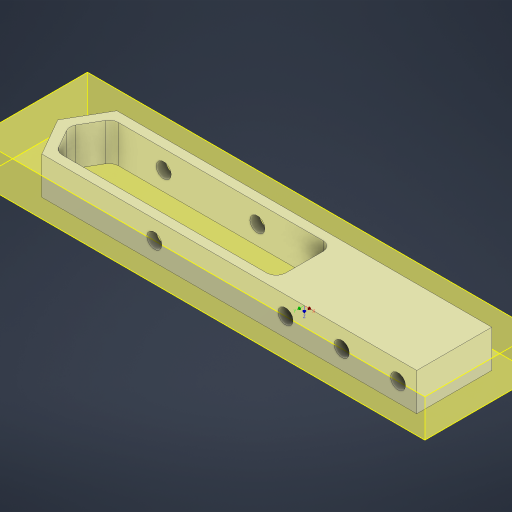
# Autodesk Inventor part: Third Baseplate Spacer
Saved by Autodesk Inventor 2023 (Build 270158000, 158)
## iProperties
Created: 2022-05-02
Part Number: Third Baseplate Spacer
Material: Generic
Document SubType Name: Modeling
Designer: FizzyApple12
Density: 1 g/cm^3
Appearance: Default
Author: FizzyApple12
Autodesk Inventor part; units mm, degrees
ref_plane "YZ Plane" through (0, 0, 0) normal (1, 0, 0) x (0, 1, 0)
ref_plane "XZ Plane" through (0, 0, 0) normal (0, 1, 0) x (-1, 0, 0)
ref_plane "XY Plane" through (0, 0, 0) normal (0, 0, 1) x (1, 0, 0)
sketch "Sketch1" plane through (0, 0, 0) normal (0, 0, 1) x (1, 0, 0)
  line L0 (0, 0) -> (50.8, 0)
  line L1 (50.8, 0) -> (50.8, 12.7)
  line L2 (50.8, 12.7) -> (0, 12.7)
  line L3 (0, 12.7) -> (0, 0)
  dimension "d0" = 50.8
  dimension "d1" = 12.7
  constraints: 8 end point, 2 parallel, 1 horizontal, 1 perpendicular
  measures "d0" distance of L2.end L1.end
  measures "d1" distance of L1.end L0.end
extrude "Extrusion1" add sketch "Sketch1" along normal blind 25.4
sketch "Sketch2" plane through (0, 0, 25.4) normal (0, 0, 1) x (1, 0, 0)
  line L0 (50.8, 12.7) -> (0, 12.7) construction
  line L1 (50.8, 0) -> (50.8, 12.7) construction
  line L2 (0, 12.7) -> (50.8, 12.7) construction
  line L3 (50.8, 12.7) -> (50.8, 6.35) construction
  line L4 (50.8, 6.35) -> (0, 6.35) construction
  line L5 (0, 6.35) -> (0, 12.7) construction
  point P0 (0, 0)
  point P1 (25.4, 6.35)
  point P2 (6.35, 6.35)
  point P3 (44.45, 6.35)
  dimension "d4" = 6.35
  dimension "d5" = 19.05
  dimension "d6" = 19.05
  constraints: 8 end point, 2 midpoint, 2 parallel, 2 point on line, 1 horizontal, 1 perpendicular
  measures "d4" distance of L2.end L3.end
  measures "d5" distance of point (6.35, 6.35) point (25.4, 6.35)
  measures "d6" distance of point (44.45, 6.35) point (25.4, 6.35)
hole "Hole1" at (25.4, 6.35, 25.4) at (6.35, 6.35, 25.4) at (44.45, 6.35, 25.4) direction (0, 0, -1) diameter 5.1054 end through all clearance for "Hex Machine Screw" size "#10" standard "Ansi Unified Screw Threads"
sketch "Sketch3" plane through (0, 0, 0) normal (-1, 0, 0) x (0, 0, 1)
  line L0 (0, 0) -> (0, 12.7) projected
  line L1 (0, 12.7) -> (25.4, 12.7) projected
  line L2 (0, 0) -> (25.4, 0)
  line L3 (25.4, 0) -> (25.4, 12.7)
  line L4 (25.4, 12.7) -> (0, 12.7)
  line L5 (0, 12.7) -> (0, 0)
  constraints: 8 end point, 2 parallel, 1 horizontal, 1 perpendicular
extrude "Extrusion2" add sketch "Sketch3" along normal blind 76.2
sketch "Sketch4" plane through (50.8, 12.7, 25.4) normal (0, 1, 0) x (1, 0, 0)
  line L0 (-127, 25.4) -> (-127, 0) projected
  line L1 (-127, 12.7) -> (-134.3323, 12.7)
  line L2 (-134.3323, 12.7) -> (-127, 0)
  line L3 (-127, 0) -> (-127, 25.4)
  line L4 (-127, 25.4) -> (-134.3323, 12.7)
  point P0 (-50.8, 25.4)
  dimension "d16" = 7.3323
  constraints: 8 end point, 1 horizontal, 1 midpoint, 1 perpendicular
  measures "d16" distance of L1.start L1.end
extrude "Extrusion3" add sketch "Sketch4" against normal up to surface (12.7 mm away)
sketch "Sketch5" plane through (50.8, 12.7, 25.4) normal (0, 1, 0) x (1, 0, 0)
  line L0 (-134.3323, 12.7) -> (-127, 0) projected
  line L1 (-127, 25.4) -> (-134.3323, 12.7) projected
  line L2 (0, 25.4) -> (-127, 25.4) projected
  line L3 (0, 0) -> (-127, 0) projected
  line L4 (0, 25.4) -> (0, 0) projected
  line L5 (-125.1669, 22.225) -> (-130.6662, 12.7)
  line L6 (-130.6662, 12.7) -> (-125.1669, 3.175)
  line L7 (-125.1669, 3.175) -> (-50.8, 3.175)
  line L8 (-50.8, 3.175) -> (-50.8, 22.225)
  line L9 (-50.8, 22.225) -> (-125.1669, 22.225)
  point P0 (-50.8, 25.4)
  dimension "d19" = 3.175
  dimension "d20" = 3.175
  dimension "d21" = 3.175
  dimension "d22" = 3.175
  dimension "d23" = 3.175
  dimension "d24" = 3.175
  dimension "d25" = 3.175
  dimension "d26" = 3.175
  dimension "d27" = 50.8
  dimension "d28" = 50.8
  constraints: 10 end point
  measures "d19" distance from line of L0 L5.end
  measures "d20" distance from line of L1 L5.end
  measures "d21" distance from line of L2 L5.start
  measures "d22" distance from line of L1 L5.start
  measures "d23" distance from line of L3 L6.end
  measures "d24" distance from line of L0 L6.end
  measures "d25" distance from line of L3 L7.end
  measures "d26" distance from line of L2 L8.end
  measures "d27" distance from line of L4 L8.end
  measures "d28" distance from line of L4 L7.end
extrude "Extrusion4" cut sketch "Sketch5" against normal through all contours L9 L8 L7 L6 L5
sketch "Sketch6" plane through (0, 0, 0) normal (0, 0, 1) x (1, 0, 0)
  line L0 (-76.2, 0) -> (-76.2, 12.7) construction
  line L1 (-76.2, 6.35) -> (50.8, 6.35) construction
  line L2 (50.8, 0) -> (50.8, 12.7) construction
  point P0 (0, 0)
  point P1 (-57.15, 6.35)
  point P2 (-25.4, 6.35)
  dimension "d31" = 31.75
  dimension "d32" = 19.05
  constraints: 2 end point, 2 midpoint, 2 point on line
  measures "d31" distance of point (-25.4, 6.35) point (-57.15, 6.35)
  measures "d32" distance from line of L0 point (-57.15, 6.35)
hole "Hole2" at (-57.15, 6.35, 0) at (-25.4, 6.35, 0) direction (0, 0, 1) diameter 5.1054 depth 8.89 clearance for "Flat Head Machine Screw (82)" size "#10" standard "Ansi Unified Screw Threads"
sketch "Sketch7" plane through (0, 0, 25.4) normal (0, 0, 1) x (1, 0, 0)
  line L0 (-76.2, 0) -> (-76.2, 12.7) construction
  line L1 (-76.2, 6.35) -> (50.8, 6.35) construction
  line L2 (50.8, 0) -> (50.8, 12.7) construction
  point P0 (0, 0)
  point P1 (-38.1, 6.35)
  dimension "d40" = 38.1
  constraints: 2 end point, 2 midpoint, 1 point on line
  measures "d40" distance from line of L0 point (-38.1, 6.35)
hole "Hole3" at (-38.1, 6.35, 25.4) direction (0, 0, -1) diameter 5.1054 depth 16.51 clearance for "Flat Head Machine Screw (82)" size "#10" standard "Ansi Unified Screw Threads"
fillet "Fillet1" radius 3.175 5 edges at (0, 6.35, 3.175) (0, 6.35, 22.225) (-74.3669, 6.35, 3.175) (-79.8662, 6.35, 12.7) (-74.3669, 6.35, 22.225)
chamfer "Chamfer1" [suppressed]
body "Solid1"
